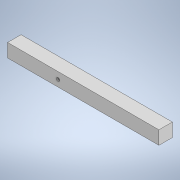
# Autodesk Inventor part: CatapultArm
Saved by Autodesk Inventor 2022.2 (Build 262287000, 287)
## iProperties
Created: 2022-01-16
Part Number: CatapultArm
Material: Generic
Document SubType Name: Modeling
Designer: robst
Density: 1 g/cm^3
Appearance: Default
Author: robst
Autodesk Inventor part; units mm, degrees
ref_plane "YZ Plane" through (0, 0, 0) normal (1, 0, 0) x (0, 1, 0)
ref_plane "XZ Plane" through (0, 0, 0) normal (0, 1, 0) x (-1, 0, 0)
ref_plane "XY Plane" through (0, 0, 0) normal (0, 0, 1) x (1, 0, 0)
sketch "Sketch2" plane through (0, 0, 0) normal (0, 0, 1) x (1, 0, 0)
  circle A0 centre (0, 0) radius 12.7
  line L0 (12.7, 0) -> (762, 0)
  line L1 (762, 0) -> (762, 50.8)
  line L2 (762, 50.8) -> (0, 50.8)
  line L3 (0, 50.8) -> (0, 12.7)
  line L4 (762, 0) -> (762, -50.8)
  line L5 (762, -50.8) -> (0, -50.8)
  line L6 (0, -50.8) -> (0, -12.7)
  line L7 (-12.7, 0) -> (-381, 0)
  line L8 (-381, 0) -> (-381, 50.8)
  line L9 (-381, 50.8) -> (0, 50.8)
  line L10 (0, 50.8) -> (0, 12.7)
  line L11 (0, -50.8) -> (0, -12.7)
  line L12 (-381, 0) -> (-381, -50.8)
  line L13 (-381, -50.8) -> (0, -50.8)
  dimension "d0" = 25.4
  dimension "d1" = 50.8
  dimension "d2" = 762
  dimension "d3" = 381
  constraints: 28 end point, 6 symmetric about line, 4 parallel, 3 point on circle, 2 horizontal, 2 perpendicular, 1 centre point, 1 coincident, 1 point on line
  measures "d0" diameter of A0
  measures "d1" distance of L0.end L1.end
  measures "d2" distance of L1.end L2.end
  measures "d3" distance of L8.end L9.end
extrude "Extrusion1" add sketch "Sketch2" along normal mid plane 101.6 contours L0 L4 L5 L6 A0 | A0 L3 L2 L1 L0 | A0 L7 L8 L9 L3 | L6 L13 L12 L7 A0
equation "\"d2\" = longDistanceFromHole"
equation "\"d3\" = shortDistanceFromHole"
equation "\"materialWidth\" = 101.6"
equation "\"shortDistanceFromHole\" = 381"
equation "\"longDistanceFromHole\" = 762"
body "Solid1"
